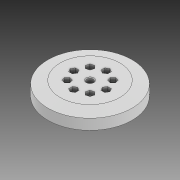
# Autodesk Inventor part: J0_DriveDisc
Saved by Autodesk Inventor 2020 (Build 240168000, 168)
## iProperties
Created: 2021-06-10
Part Number: J0_DriveDisc
Material: Generic
Document SubType Name: Modeling
Designer: DDeGo
Density: 1 g/cm^3
Appearance: Default
Author: DDeGo
Autodesk Inventor part; units mm, degrees
ref_plane "YZ Plane" through (0, 0, 0) normal (1, 0, 0) x (0, 1, 0)
ref_plane "XZ Plane" through (0, 0, 0) normal (0, 1, 0) x (-1, 0, 0)
ref_plane "XY Plane" through (0, 0, 0) normal (0, 0, 1) x (1, 0, 0)
sketch "Sketch1" plane through (0, 0, 0) normal (0, 0, 1) x (1, 0, 0)
  line L0 (-34, 0) -> (-27, 0) construction
  line L1 (-34, 0) -> (-34, 3.5) construction
  line L2 (-34, 5) -> (-48.1998, 5)
  line L3 (-48.1998, 5) -> (-48.1998, 1)
  line L4 (-48.1998, 1) -> (-52, 1)
  line L5 (-52, 1) -> (-52, 14)
  line L6 (-52, 14) -> (-37, 18)
  line L7 (0, 10) -> (0, 0)
  line L8 (-37, 18) -> (-4, 18)
  line L9 (0, 10) -> (-4, 10)
  line L10 (-4, 10) -> (-4, 18)
  line L11 (-34, 3.5) -> (-27, 3.5)
  line L12 (-27, 3.5) -> (-27, 0)
  line L13 (-34, 3.5) -> (-34, 5)
  line L14 (-27, 0) -> (-24.9, 0)
  line L15 (-24.9, 0) -> (-24.9, -3)
  line L16 (-24.9, -3) -> (0, -3)
  line L17 (0, -3) -> (0, 0)
  line L18 (-24.9, 0) -> (0, 0) construction
  dimension "d8" = 4
  dimension "d9" = 14.1998
  dimension "d10" = 34
  dimension "d11" = 5
  dimension "d13" = 13
  dimension "d14" = 15
  dimension "d15" = 52
  dimension "d21" = 13
  dimension "d37" = 4
  dimension "d38" = 8
  dimension "d42" = 27
  dimension "d43" = 3.5
  dimension "d44" = 3
  dimension "d45" = 24.9
  constraints: 39 end point, 10 perpendicular, 4 horizontal, 3 vertical, 1 coincident
  measures "d8" distance between parallel lines of L2 L4
  measures "d9" distance between parallel lines of L1 L3
  measures "d10" distance between parallel lines of L7 L1
  measures "d11" distance between parallel lines of L0 L2
  measures "d13" distance of L5.start L5.end
  measures "d14" horizontal distance of L6.end L5.end
  measures "d15" distance between parallel lines of L7 L5
  measures "d21" distance between parallel lines of L8 L2
  measures "d37" distance between parallel lines of L7 L10
  measures "d38" distance of L9.end L8.end
  measures "d42" distance between parallel lines of L7 L12
  measures "d43" distance of L11.end L0.end
  measures "d44" distance of L14.end L15.end
  measures "d45" distance between parallel lines of L17 L15
revolve "Revolution1" add sketch "Sketch1" angle 360 about axis through (0, 10, 0) along (0, -1, 0)
sketch "Sketch2" plane through (0, 0, 0) normal (0, -1, 0) x (1, 0, 0)
  circle A0 centre (0, 20) radius 2.75
  line L0 (0, 20) -> (0, 0) construction
  line L1 (-14.1421, 14.1421) -> (0, 0) construction
  circle A1 centre (-14.1421, 14.1421) radius 2.75
  line L2 (-20, 0) -> (0, 0) construction
  circle A2 centre (-20, 0) radius 2.75
  line L3 (-14.1421, -14.1421) -> (0, 0) construction
  circle A3 centre (-14.1421, -14.1421) radius 2.75
  line L4 (0, -20) -> (0, 0) construction
  circle A4 centre (0, -20) radius 2.75
  line L5 (14.1421, -14.1421) -> (0, 0) construction
  circle A5 centre (14.1421, -14.1421) radius 2.75
  line L6 (20, 0) -> (0, 0) construction
  circle A6 centre (20, 0) radius 2.75
  line L7 (14.1421, 14.1421) -> (0, 0) construction
  circle A7 centre (14.1421, 14.1421) radius 2.75
  dimension "d22" = 20
  dimension "d23" = 5.5
  dimension "d26" = 360
  constraints: 16 end point, 8 centre point, 2 coincident, 1 vertical, 31 other
  measures "d22" distance of L0.start L0.end
  measures "d23" diameter of A0
extrude "Extrusion1" cut sketch "Sketch2" against normal through all both and the other way through all
sketch "Sketch3" plane through (0, 18, 0) normal (0, 1, 0) x (1, 0, 0)
  line L0 (0, -15.2657) -> (4.1, -17.6329)
  line L1 (4.1, -17.6329) -> (4.1, -22.3671)
  line L2 (4.1, -22.3671) -> (0, -24.7343)
  line L3 (0, -24.7343) -> (-4.1, -22.3671)
  line L4 (-4.1, -22.3671) -> (-4.1, -17.6329)
  line L5 (-4.1, -17.6329) -> (0, -15.2657)
  line L6 (10.7945, -10.7945) -> (15.3675, -9.5692)
  line L7 (15.3675, -9.5692) -> (18.7151, -12.9168)
  line L8 (18.7151, -12.9168) -> (17.4898, -17.4898)
  line L9 (17.4898, -17.4898) -> (12.9168, -18.7151)
  line L10 (12.9168, -18.7151) -> (9.5692, -15.3675)
  line L11 (9.5692, -15.3675) -> (10.7945, -10.7945)
  line L12 (15.2657, 0) -> (17.6329, 4.1)
  line L13 (17.6329, 4.1) -> (22.3671, 4.1)
  line L14 (22.3671, 4.1) -> (24.7343, 0)
  line L15 (24.7343, 0) -> (22.3671, -4.1)
  line L16 (22.3671, -4.1) -> (17.6329, -4.1)
  line L17 (17.6329, -4.1) -> (15.2657, 0)
  line L18 (10.7945, 10.7945) -> (9.5692, 15.3675)
  line L19 (9.5692, 15.3675) -> (12.9168, 18.7151)
  line L20 (12.9168, 18.7151) -> (17.4898, 17.4898)
  line L21 (17.4898, 17.4898) -> (18.7151, 12.9168)
  line L22 (18.7151, 12.9168) -> (15.3675, 9.5692)
  line L23 (15.3675, 9.5692) -> (10.7945, 10.7945)
  line L24 (0, 15.2657) -> (-4.1, 17.6329)
  line L25 (-4.1, 17.6329) -> (-4.1, 22.3671)
  line L26 (-4.1, 22.3671) -> (0, 24.7343)
  line L27 (0, 24.7343) -> (4.1, 22.3671)
  line L28 (4.1, 22.3671) -> (4.1, 17.6329)
  line L29 (4.1, 17.6329) -> (0, 15.2657)
  line L30 (-10.7945, 10.7945) -> (-15.3675, 9.5692)
  line L31 (-15.3675, 9.5692) -> (-18.7151, 12.9168)
  line L32 (-18.7151, 12.9168) -> (-17.4898, 17.4898)
  line L33 (-17.4898, 17.4898) -> (-12.9168, 18.7151)
  line L34 (-12.9168, 18.7151) -> (-9.5692, 15.3675)
  line L35 (-9.5692, 15.3675) -> (-10.7945, 10.7945)
  line L36 (-15.2657, 0) -> (-17.6329, -4.1)
  line L37 (-17.6329, -4.1) -> (-22.3671, -4.1)
  line L38 (-22.3671, -4.1) -> (-24.7343, 0)
  line L39 (-24.7343, 0) -> (-22.3671, 4.1)
  line L40 (-22.3671, 4.1) -> (-17.6329, 4.1)
  line L41 (-17.6329, 4.1) -> (-15.2657, 0)
  line L42 (-10.7945, -10.7945) -> (-9.5692, -15.3675)
  line L43 (-9.5692, -15.3675) -> (-12.9168, -18.7151)
  line L44 (-12.9168, -18.7151) -> (-17.4898, -17.4898)
  line L45 (-17.4898, -17.4898) -> (-18.7151, -12.9168)
  line L46 (-18.7151, -12.9168) -> (-15.3675, -9.5692)
  line L47 (-15.3675, -9.5692) -> (-10.7945, -10.7945)
  point P0 (0, 0)
  point P1 (0, -20)
  point P2 (0, -20)
  point P3 (14.1421, -14.1421)
  point P4 (14.1421, -14.1421)
  point P5 (20, 0)
  point P6 (20, 0)
  point P7 (14.1421, 14.1421)
  point P8 (14.1421, 14.1421)
  point P9 (0, 20)
  point P10 (0, 20)
  point P11 (-14.1421, 14.1421)
  point P12 (-14.1421, 14.1421)
  point P13 (-20, 0)
  point P14 (-20, 0)
  point P15 (-14.1421, -14.1421)
  point P16 (-14.1421, -14.1421)
  dimension "d30" = 8.2
  dimension "d33" = 360
  constraints: 96 end point, 8 coincident, 1 vertical, 126 other
  measures "d30" distance between parallel lines of L4 L1
extrude "Extrusion2" cut sketch "Sketch3" against normal blind 5
chamfer "Chamfer1" distance 1 angle 45 1 edges at (4, 18, 0)
body "Solid1"
